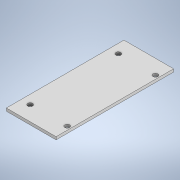
# Autodesk Inventor part: PosiblePlaca
Saved by Autodesk Inventor 2021 (Build 250183000, 183)
## iProperties
Created: 2021-10-29
Part Number: PosiblePlaca
Material: Genérico
Document SubType Name: Chapa
Designer: Juan Camilo
Density: 1 g/cm^3
Sheet Metal Rule: Por defecto_mm
Appearance: Valor por defecto
Author: Juan Camilo
Autodesk Inventor part; units mm, degrees
ref_plane "YZ Plane" through (0, 0, 0) normal (1, 0, 0) x (0, 1, 0)
ref_plane "XZ Plane" through (0, 0, 0) normal (0, 1, 0) x (-1, 0, 0)
ref_plane "XY Plane" through (0, 0, 0) normal (0, 0, 1) x (1, 0, 0)
sketch "Boceto1" plane through (0, 0, 0) normal (0, 1, 0) x (-1, 0, 0)
  line L0 (8.0156, 39.7394) -> (-27.4844, 39.7394)
  line L1 (-27.4844, 39.7394) -> (-27.4844, -44.2606)
  line L2 (-27.4844, -44.2606) -> (8.0156, -44.2606)
  line L3 (8.0156, -44.2606) -> (8.0156, 39.7394)
  circle A0 centre (1.5156, 29.2394) radius 1.75
  circle A1 centre (-24.9844, 29.2394) radius 1.75
  line L4 (8.0156, -2.2606) -> (-27.4844, -2.2606)
  circle A2 centre (1.5156, -33.7606) radius 1.75
  circle A3 centre (-24.9844, -33.7606) radius 1.75
  point P0 (0, 0)
  dimension "d0" = 84
  dimension "d1" = 35.5
  dimension "d2" = 3.5
  dimension "d3" = 6.5
  dimension "d4" = 10.5
  dimension "d5" = 3.5
  dimension "d6" = 26.5
  dimension "d7" = 84
  dimension "d8" = 84
  dimension "d9" = 63
  constraints: 10 end point, 4 centre point, 2 midpoint, 2 parallel, 2 perpendicular, 2 symmetric about line, 1 horizontal, 2 other
  measures "d0" distance of L2.end L0.start
  measures "d1" distance between parallel lines of L1 L3
  measures "d2" diameter of A0
  measures "d3" distance from line of L3 A0.centre
  measures "d4" distance from line of L0 A0.centre
  measures "d5" diameter of A1
  measures "d6" distance of A0.centre A1.centre
  measures "d7" diameter of L0 L4
  measures "d8" diameter of L2 L4
  measures "d9" distance of A2.centre A0.centre
extrude "Extrusión1" add sketch "Boceto1" along normal blind 2
equation "\"Radio_pliegue\" = Grosor"
equation "\"Anchura_desahogo_plegado\" = Grosor"
equation "\"Profundidad_desahogo_plegado\" = 0.5 * Grosor"
equation "\"Tamaño_destalonado\" = 4 * Grosor"
equation "\"Remanente_mínimo\" = 2 * Grosor"
equation "\"Radiodetransición\" = Radio_pliegue"
equation "\"Tamaño_de_radio_de_Jacobi\" = Radio_pliegue"
equation "\"TamañoSeparación\" = Grosor"
equation "\"Grosor\" = 0.5"
